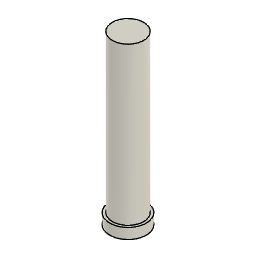
Axle (Autodesk Fusion 360 design; units mm, degrees)
Autodesk Fusion 360 part; units mm, degrees
sketch "Esboço1" plane through (0, 0, 0) normal (0, 0, 1) x (1, 0, 0)
  circle A0 centre (10, 5) radius 3
  circle A1 centre (10, 5) radius 3.5
  dimension "d1" = 6
  dimension "d2" = 7
  constraint concentric A0 A1
  measures "d1" diameter of A0
  measures "d2" diameter of A1
extrude "Extrusão1" add sketch "Esboço1" along normal blind 31 contours A0
extrude "Extrusão2" add sketch "Esboço1" along normal blind 1
extrude "Extrusão3" add sketch "Esboço1" against normal blind 1 contours A0 | A1
